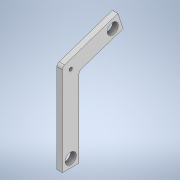
# Autodesk Inventor part: bogie1
Saved by Autodesk Inventor 2020 (Build 240168000, 168)
## iProperties
Created: 2020-05-30
Part Number: bogie1
Material: Generic
Document SubType Name: Modeling
Designer: Manish
Density: 1 g/cm^3
Appearance: Default
Author: Manish
Autodesk Inventor part; units mm, degrees
ref_plane "YZ Plane" through (0, 0, 0) normal (1, 0, 0) x (0, 1, 0)
ref_plane "XZ Plane" through (0, 0, 0) normal (0, 1, 0) x (-1, 0, 0)
ref_plane "XY Plane" through (0, 0, 0) normal (0, 0, 1) x (1, 0, 0)
sketch "Sketch1" plane through (0, 0, 0) normal (1, 0, 0) x (0, 1, 0)
  circle A0 centre (0, 0) radius 3
  line L0 (6.4648, 15) -> (-155, 15)
  line L1 (-155, 15) -> (-155, -15)
  line L2 (-155, -15) -> (-15.0845, -15)
  line L3 (15, -15) -> (15, 15)
  line L4 (-9.3985, -19.0843) -> (16.2364, -95.1689)
  line L5 (16.2364, -95.1689) -> (44.6661, -85.5902)
  line L6 (44.6661, -85.5902) -> (12.1507, 10.9157)
  line L7 (9.5442, 18.6521) -> (-18.8856, 9.0734)
  arc A1 (-9.3985, -19.0843) -> (-15.0845, -15) centre (-15.0845, -21) ccw
  arc A2 (12.1507, 10.9157) -> (6.4648, 15) centre (6.4648, 9) ccw
  circle A3 centre (-140, 0) radius 10
  circle A4 centre (-140, 0) radius 3
  circle A5 centre (25.6619, -76.1647) radius 10
  dimension "d0" = 6
  dimension "d1" = 170
  dimension "d2" = 30
  dimension "d3" = 110
  dimension "d6" = 108.62
  dimension "d7" = 15
  dimension "d8" = 15
  dimension "d9" = 6
  dimension "d10" = 20
  dimension "d11" = 6
  dimension "d12" = 15
  dimension "d13" = 20
  constraints: 16 end point, 6 centre point, 4 parallel, 4 point on circle, 4 point on line, 4 tangent, 3 coincident, 2 perpendicular, 1 equal radius, 1 horizontal
  measures "d0" diameter of A0
  measures "d1" distance of L3.start L1.end
  measures "d2" distance of L1.end L0.end
  measures "d3" distance of L7.start L5.end
  measures "d6" angle of L4 L2
  measures "d7" distance from line of point (0, 0) L6
  measures "d8" distance from line of L2 point (0, 0)
  measures "d9" radius of A1
  measures "d10" diameter of A3
  measures "d11" diameter of A4
  measures "d12" distance from line of L5 point (25.662, -76.165)
  measures "d13" diameter of A5
extrude "Extrusion1" add sketch "Sketch1" along normal blind 10 contours A2 L6 L5 L4 A1 L2 L1 L0
body "Solid1"
